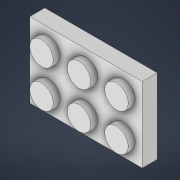
# Autodesk Inventor part: 0401_練習
Saved by Autodesk Inventor 2022 (Build 260153000, 153)
## iProperties
Created: 2022-04-01
Part Number: 0401_練習
Material: 一般
Document SubType Name: Modeling
Designer: User
Density: 1 g/cm^3
Appearance: 預設
Author: User
Autodesk Inventor part; units mm, degrees
ref_plane "YZ Plane" through (0, 0, 0) normal (1, 0, 0) x (0, 1, 0)
ref_plane "XZ Plane" through (0, 0, 0) normal (0, 1, 0) x (-1, 0, 0)
ref_plane "XY Plane" through (0, 0, 0) normal (0, 0, 1) x (1, 0, 0)
sketch "草圖1" plane through (0, 0, 0) normal (0, 1, 0) x (-1, 0, 0)
  line L0 (0, 0) -> (-16, 0)
  line L1 (-16, 0) -> (-16, -24)
  line L2 (-16, -24) -> (0, -24)
  line L3 (0, -24) -> (0, 0)
  dimension "長" = 16
  dimension "寬" = 24
  constraints: 8 end point, 2 parallel, 1 horizontal, 1 perpendicular
  measures "長" distance of L2.end L1.end
  measures "寬" distance of L1.end L0.end
extrude "樂高擠出" add sketch "草圖1" against normal blind 3.2
sketch "草圖2" plane through (0, 0, 0) normal (0, 1, 0) x (-1, 0, 0)
  circle A0 centre (-12, -4) radius 2.5
  line L0 (-16, 0) -> (-16, -24) projected
  line L1 (0, 0) -> (-16, 0) projected
  dimension "d4" = 5
  dimension "d5" = 4
  dimension "d6" = 4
  constraints: 1 centre point
  measures "d4" diameter of A0
  measures "d5" distance from line of L0 A0.centre
  measures "d6" distance from line of L1 A0.centre
extrude "圓柱擠出" add sketch "草圖2" along normal blind 1.5
pattern_linear "頂部圓柱" count 3 spacing 8 along (0, 0, -1) count 2 spacing 8 along (-1, 0, 0) of "圓柱擠出"
shell "薄殼2" thickness 1 removed faces 1 at (10.666667, -3.2, -16)
sketch "草圖6" plane through (1, -1, -1) normal (0, -1, 0) x (1, 0, 0)
  circle A0 centre (3, -19) radius 1.5
  circle A1 centre (3, -11) radius 1.5
  circle A2 centre (3, -3) radius 1.5
  circle A3 centre (11, -19) radius 1.5
  circle A4 centre (11, -11) radius 1.5
  circle A5 centre (11, -3) radius 1.5
  line L0 (14, 0) -> (14, -22)
  line L1 (0, 0) -> (14, 0)
  line L2 (0, -22) -> (0, 0)
  line L3 (14, -22) -> (0, -22)
  circle A6 centre (7, -7) radius 3.156854
  circle A7 centre (11, -11) radius 2.5
  circle A8 centre (11, -3) radius 2.5
  circle A9 centre (3, -3) radius 2.5
  circle A10 centre (7, -7) radius 2.156854
  point P0 (-1, 1)
  dimension "d41" = 1
  constraints: 3 tangent, 2 centre point
  measures "d41" radial gap between concentric circles of A6 A10
extrude "擠出7" add sketch "草圖6" along normal up to surface (2.2 mm away) contours A6
pattern_linear "矩形陣列3" count 2 spacing 8 along (0, 0, -1) of "擠出7"
